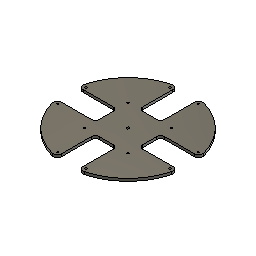
Omni-robot-JSC (Autodesk Fusion 360 archive; units mm, degrees)
design "BottomBody"
Autodesk Fusion 360 part; units mm, degrees
sketch "Sketch1" plane through (0, 0, 0) normal (0, 1, 0) x (1, 0, 0)
  circle A0 centre (0, 0) radius 152.4
  dimension "d1" = 304.8
  measures "d1" diameter of A0
extrude "Extrude1" add sketch "Sketch1" along normal blind 6.35
sketch "Sketch4" plane through (0, 6.35, 0) normal (0, 1, 0) x (-1, 0, 0)
  circle A0 centre (0, 0) radius 152.4
  circle A1 centre (0, 0) radius 3.175
  dimension "d17" = 6.35
  measures "d17" diameter of A1
extrude "Extrude3" cut sketch "Sketch4" against normal blind 63.5 contours A1
sketch "Sketch6" plane through (0, 0, 0) normal (0, -1, 0) x (1, 0, 0)
  circle A0 centre (0, 0) radius 3.175
  circle A1 centre (0, 0) radius 152.4
  circle A2 centre (0, 0) radius 142.875 construction
  circle A3 centre (-34.925, 138.5406) radius 2.159
  circle A4 centre (34.925, 138.5406) radius 2.159
  line L0 (0, 0) -> (0, 160.02) construction
  circle A5 centre (-138.5406, -34.925) radius 2.159
  circle A6 centre (-138.5406, 34.925) radius 2.159
  circle A7 centre (34.925, -138.5406) radius 2.159
  circle A8 centre (-34.925, -138.5406) radius 2.159
  circle A9 centre (138.5406, 34.925) radius 2.159
  circle A10 centre (138.5406, -34.925) radius 2.159
  dimension "d60" = 9.525
  dimension "d61" = 4.318
  dimension "d62" = 4.318
  dimension "d63" = 34.925
  dimension "d64" = 34.925
  dimension "d66" = 360
  measures "d60" distance of A1 A2
  measures "d61" diameter of A3
  measures "d62" diameter of A4
extrude "Extrude4" cut sketch "Sketch6" against normal through all contours A3 | A4 | A5 | A6 | A7 | A8 | A9 | A10
sketch "Sketch7" plane through (0, 0, 0) normal (0, -1, 0) x (1, 0, 0)
  circle A0 centre (138.5406, 34.925) radius 2.159
  circle A1 centre (-138.5406, -34.925) radius 2.159
  circle A2 centre (34.925, -138.5406) radius 2.159
  circle A3 centre (34.925, 138.5406) radius 2.159
  circle A4 centre (138.5406, -34.925) radius 2.159
  circle A5 centre (-138.5406, 34.925) radius 2.159
  circle A6 centre (-34.925, -138.5406) radius 2.159
  circle A7 centre (-34.925, 138.5406) radius 2.159
  circle A8 centre (0, 0) radius 3.175
  circle A9 centre (0, 0) radius 152.4
  line L0 (0, 0) -> (53.8815, 53.8815) construction
  line L1 (0, 0) -> (76.2, 0) construction
  circle A10 centre (0, 0) radius 76.2 construction
  circle A11 centre (53.8815, 53.8815) radius 2.159
  circle A12 centre (-53.8815, 53.8815) radius 2.159
  circle A13 centre (-53.8815, -53.8815) radius 2.159
  circle A14 centre (53.8815, -53.8815) radius 2.159
  dimension "d68" = 45
  dimension "d69" = 76.2
  dimension "d70" = 73.025
  dimension "d71" = 4.318
  dimension "d73" = 360
  measures "d68" angle of L0 L1
  measures "d70" distance of A8 A10
  measures "d71" diameter of A11
extrude "Extrude5" cut sketch "Sketch7" against normal through all contours A11 | A12 | A13 | A14
sketch "Sketch3" plane through (0, 0, 0) normal (0, -1, 0) x (1, 0, 0)
  circle A0 centre (0, 0) radius 152.4
  line L0 (0, 0) -> (0, -214.9258) construction
  line L1 (14.986, -57.15) -> (-14.986, -57.15) construction
  line L2 (-14.986, -57.15) -> (-14.986, -247.65) construction
  line L3 (-14.986, -247.65) -> (14.986, -247.65) construction
  line L4 (14.986, -247.65) -> (14.986, -57.15) construction
  line L5 (14.986, -57.15) -> (-14.986, -247.65) construction
  line L6 (-14.986, -57.15) -> (14.986, -247.65) construction
  line L7 (-14.986, -68.58) -> (14.986, -68.58) construction
  line L8 (-14.986, -95.25) -> (14.986, -95.25) construction
  line L9 (26.9875, -250.825) -> (-26.9875, -250.825)
  line L10 (-26.9875, -250.825) -> (-26.9875, -53.975)
  line L11 (-26.9875, -53.975) -> (26.9875, -53.975)
  line L12 (26.9875, -53.975) -> (26.9875, -250.825)
  line L13 (26.9875, -250.825) -> (-26.9875, -53.975) construction
  line L14 (-26.9875, -250.825) -> (26.9875, -53.975) construction
  circle A1 centre (-53.8815, 53.8815) radius 2.159
  circle A2 centre (-53.8815, -53.8815) radius 2.159
  circle A3 centre (53.8815, 53.8815) radius 2.159
  circle A4 centre (53.8815, -53.8815) radius 2.159
  circle A5 centre (138.5406, 34.925) radius 2.159
  circle A6 centre (-138.5406, -34.925) radius 2.159
  circle A7 centre (34.925, -138.5406) radius 2.159
  circle A8 centre (34.925, 138.5406) radius 2.159
  circle A9 centre (138.5406, -34.925) radius 2.159
  circle A10 centre (-138.5406, 34.925) radius 2.159
  circle A11 centre (-34.925, -138.5406) radius 2.159
  circle A12 centre (-34.925, 138.5406) radius 2.159
  circle A13 centre (0, 0) radius 3.175
  dimension "d5" = 190.5
  dimension "d6" = 29.972
  dimension "d7" = 11.43
  dimension "d8" = 38.1
  dimension "d76" = 53.975
  dimension "d77" = 196.85
  measures "d7" distance of L1 L7
  measures "d8" distance of L1 L8
extrude "Extrude6" cut sketch "Sketch3" against normal blind 88.9 contours A0 L10 L11 L12 picked at (-3.0127, -86.6939)
fillet "Fillet1" radius 9.525 4 edges at (-26.9875, 3.175, -149.9914) (-26.9875, 3.175, -53.975) (26.9875, 3.175, -53.975) (26.9875, 3.175, -149.9914)
pattern_circular "C-Pattern3" count 4 over 360 about axis through (0, 1.75, 0) along (0, 1, 0) of "Extrude6", "Fillet1"
equation "d5 = ( 3.75 * 2 ) * 1 in"
equation "d70 = 1 in + 1.875 in"

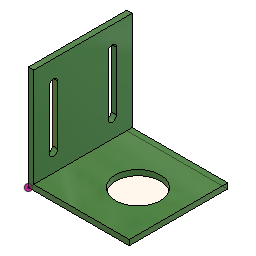
design "brackets"
Autodesk Fusion 360 part; units mm, degrees
sketch "Sketch2" plane through (0, 0, 0) normal (0, 1, 0) x (1, 0, 0)
  line L0 (0, 0) -> (51.562, 0)
  line L1 (51.562, 0) -> (51.562, 50.292)
  line L2 (51.562, 50.292) -> (0, 50.292)
  line L3 (0, 50.292) -> (0, 0)
  dimension "d1" = 51.562
  dimension "d2" = 50.292
extrude "Extrude1" add sketch "Sketch2" along normal blind 2.7432
sketch "Sketch3" plane through (0, 0, 0) normal (-1, 0, 0) x (0, 0, 1)
  line L0 (-50.292, 0) -> (0, 0)
  line L1 (0, 0) -> (0, 2.7432)
  line L2 (0, 2.7432) -> (-50.292, 2.7432)
  line L3 (-50.292, 2.7432) -> (-50.292, 0)
  line L4 (-50.292, 0) -> (0, 0)
  line L5 (0, 0) -> (0, 53.34)
  line L6 (0, 53.34) -> (-50.292, 53.34)
  line L7 (-50.292, 53.34) -> (-50.292, 0)
  dimension "d5" = 53.34
  measures "d5" distance of L4 L6
extrude "Extrude2" add sketch "Sketch3" against normal blind 2.7432 contours L2 L5 L6 L7
hole "Hole1" at (30.861, 0, -25.146) direction (0, 1, 0) diameter 22.86 depth 22.86 tip angle 118
sketch "Sketch4" plane through (0, 0, 0) normal (-1, 0, 0) x (0, 0, 1)
  line L0 (-50.292, 0) -> (0, 0)
  line L1 (0, 0) -> (0, 53.34)
  line L2 (0, 53.34) -> (-50.292, 53.34)
  line L3 (-50.292, 53.34) -> (-50.292, 0)
  line L4 (-25.146, 0) -> (-25.146, 53.34) construction
  line L5 (-12.319, 44.45) -> (-8.001, 44.45)
  line L6 (-8.001, 44.45) -> (-8.001, 10.16)
  line L7 (-8.001, 10.16) -> (-12.319, 10.16)
  line L8 (-12.319, 10.16) -> (-12.319, 44.45)
  line L9 (-37.973, 10.16) -> (-37.973, 44.45)
  line L10 (-37.973, 44.45) -> (-42.291, 44.45)
  line L11 (-42.291, 44.45) -> (-42.291, 10.16)
  line L12 (-42.291, 10.16) -> (-37.973, 10.16)
  dimension "d13" = 4.318
  dimension "d14" = 34.29
  dimension "d15" = 12.827
  dimension "d16" = 8.89
  measures "d15" distance of L4 L8
  measures "d16" distance of L2 L5
extrude "Extrude3" cut sketch "Sketch4" against normal through all contours L5 L6 L7 L8 | L9 L10 L11 L12
sketch "Sketch5" plane through (0, 0, -12.319) normal (0, 0, 1) x (1, 0, 0)
  line L0 (2.7432, 10.16) -> (2.7432, 44.45)
  line L1 (2.7432, 44.45) -> (0, 44.45)
  line L2 (0, 44.45) -> (0, 10.16)
  line L3 (0, 10.16) -> (2.7432, 10.16)
fillet "Fillet1" radius 2.159 8 edges at (1.3716, 44.45, -12.319) (1.3716, 44.45, -8.001) (1.3716, 10.16, -12.319) (1.3716, 10.16, -8.001) (1.3716, 10.16, -37.973) (1.3716, 10.16, -42.291) (1.3716, 44.45, -37.973) (1.3716, 44.45, -42.291)
equation "d11 = ( 1.98 / 2 ) * 1 in"
equation "d18 = ( 0.17 / 2 ) * 1 in"
